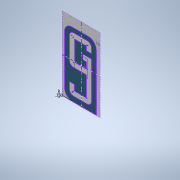
# Autodesk Inventor part: Part2
Saved by Autodesk Inventor 2021 (Build 250183000, 183)
## iProperties
Created: 2022-05-21
Part Number: Part2
Material: Generic
Document SubType Name: Modeling
Designer: cmzgt
Density: 1 g/cm^3
Appearance: Default
Author: cmzgt
Autodesk Inventor part; units mm, degrees
ref_plane "YZ Plane" through (0, 0, 0) normal (1, 0, 0) x (0, 1, 0)
ref_plane "XZ Plane" through (0, 0, 0) normal (0, 1, 0) x (-1, 0, 0)
ref_plane "XY Plane" through (0, 0, 0) normal (0, 0, 1) x (1, 0, 0)
sketch "Sketch1" plane through (0, 0, 0) normal (0, 0, 1) x (1, 0, 0)
  line L0 (76.2, -101.6) -> (-76.2, -101.6)
  line L1 (-76.2, -101.6) -> (-76.2, 101.6)
  line L2 (-76.2, 101.6) -> (76.2, 101.6)
  line L3 (76.2, 101.6) -> (76.2, -101.6)
  line L4 (76.2, -101.6) -> (-76.2, 101.6) construction
  line L5 (-76.2, -101.6) -> (76.2, 101.6) construction
  point P0 (0, 0)
  dimension "d0" = 152.4
  dimension "d1" = 203.2
  constraints: 12 end point, 2 midpoint, 2 parallel, 1 horizontal, 1 perpendicular
  measures "d0" distance of L1.end L2.end
  measures "d1" distance of L0.end L1.end
extrude "Extrusion1" add sketch "Sketch1" along normal blind 25.4
sketch "Sketch2" plane through (0, 0, 25.4) normal (0, 0, 1) x (1, 0, 0)
  line L0 (-226.9738, 447.9746) -> (224.5353, 447.9746) construction
  line L1 (224.5353, 447.9746) -> (224.5353, -428.4841) construction
  line L2 (224.5353, -428.4841) -> (-226.9738, -428.4841) construction
  line L3 (-226.9738, -428.4841) -> (-226.9738, 447.9746) construction
  line L4 (175.8473, -419.5941) -> (175.8473, 245.0143)
  arc A0 (175.8473, 245.0143) -> (81.7255, 339.136) centre (81.7255, 245.0143) ccw
  line L5 (-226.9738, 0) -> (224.5353, 0)
  line L6 (81.7255, 339.136) -> (-0.7651, 339.136)
  line L7 (-1.2193, 447.9746) -> (-1.2193, -428.4841)
  line L8 (-0.7651, 339.136) -> (-109.9973, 339.136)
  line L9 (-197.5103, -325.9614) -> (-197.5103, 251.623)
  arc A1 (-109.9973, 339.136) -> (-197.5103, 251.623) centre (-109.9973, 251.623) ccw
  line L10 (175.8473, -419.5941) -> (-103.8776, -419.5941)
  arc A2 (-197.5103, -325.9614) -> (-103.8776, -419.5941) centre (-103.8776, -325.9614) ccw
  line L11 (60.5127, 66.1602) -> (15.8186, 66.1602)
  line L12 (15.8186, 66.1602) -> (15.8186, 127.3205)
  line L13 (15.8186, 127.3205) -> (124.6599, 127.3205)
  line L14 (124.6599, 127.3205) -> (124.6599, -305.458)
  line L15 (60.5127, 66.1602) -> (60.5127, -6.4131)
  line L16 (60.5127, -6.4131) -> (-76.9699, -6.4131)
  line L17 (-76.9699, -6.4131) -> (-76.9699, 229.6915)
  line L18 (-76.9699, 229.6915) -> (60.1108, 229.6915)
  line L19 (60.1108, 229.6915) -> (60.1108, 180.1667)
  line L20 (60.1108, 180.1667) -> (122.1436, 180.1667)
  line L21 (122.1436, 180.1667) -> (122.1436, 238.418)
  arc A3 (122.1436, 238.418) -> (69.7165, 290.8451) centre (69.7165, 238.418) ccw
  line L22 (69.7165, 290.8451) -> (-92.3667, 290.8451)
  arc A4 (-92.3667, 290.8451) -> (-141.7279, 241.4839) centre (-92.3667, 241.4839) ccw
  line L23 (-141.7279, 241.4839) -> (-141.7279, -27.6599)
  arc A5 (-141.7279, -27.6599) -> (-93.4193, -67.8148) centre (-89.1074, -13.4909) ccw
  line L24 (-93.4193, -67.8148) -> (58.494, -67.8148)
  line L25 (58.494, -67.8148) -> (58.494, -301.6299)
  line L26 (58.494, -301.6299) -> (-80.5428, -301.6299)
  line L27 (-80.5428, -301.6299) -> (-80.5428, -234.1224)
  line L28 (-80.5428, -234.1224) -> (-141.7279, -234.1224)
  line L29 (-141.7279, -234.1224) -> (-141.7279, -313.9932)
  arc A6 (-141.7279, -313.9932) -> (-93.2829, -362.4382) centre (-93.2829, -313.9932) ccw
  line L30 (-93.2829, -362.4382) -> (67.6797, -362.4382)
  arc A7 (67.6797, -362.4382) -> (124.6599, -305.458) centre (67.6797, -305.458) ccw
  line L31 (-141.7279, 241.4839) -> (-141.7279, 241.4839)
  point P0 (0, 0)
  dimension "d13" = 8.89
  constraints: 56 end point, 17 point on circle, 15 tangent, 14 perpendicular, 8 centre point, 7 horizontal, 3 vertical, 2 midpoint, 2 parallel, 2 point on line, 2 other
  measures "d13" distance between parallel lines of L2 L10
body "Solid1"
